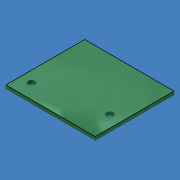
# Autodesk Inventor part: Spike PCB
Saved by Autodesk Inventor 2012 (Build 160160000, 160)
## iProperties
Shininess: 64.0
Length Units: 11269
Angle Units: 11279
Time Units: 11290
Mass Units: 11283
Length Display Precision: 3
Angle Display Precision: 2
Compacted: True
Part Number: Spike PCB
Document SubType Name: Modeling
Created: 2005-12-31
Material: Phenolic
Designer: Owner
Density: 1 g/cm^3
Density: 0.0
Volumn: 0.0
Area: 0.0
PropertySet Name: Model Information
Control State: 0
Master: False
Checked Out: False
Author: Owner
Autodesk Inventor part; units mm, degrees
ref_plane "YZ Plane" through (0, 0, 0) normal (1, 0, 0) x (0, 1, 0)
ref_plane "XZ Plane" through (0, 0, 0) normal (0, 1, 0) x (-1, 0, 0)
ref_plane "XY Plane" through (0, 0, 0) normal (0, 0, 1) x (1, 0, 0)
sketch "Sketch1" plane through (0, 0, 0) normal (0, 0, 1) x (1, 0, 0)
  line L0 (-21, 18.5) -> (21, 18.5)
  line L1 (21, 18.5) -> (21, -18.5)
  line L2 (21, -18.5) -> (-21, -18.5)
  line L3 (-21, -18.5) -> (-21, 18.5)
  line L4 (0, 0) -> (0, 18.5) construction
  line L5 (0, 0) -> (0, -18.5) construction
  line L6 (0, 0) -> (21, 0) construction
  line L7 (0, 0) -> (-21, 0) construction
  dimension "d0" = 42
  dimension "d1" = 37
  constraints: 16 end point, 4 midpoint, 3 horizontal, 2 collinear, 2 parallel, 1 perpendicular, 1 other
  measures "d0" distance of L0.start L0.end
  measures "d1" distance of L0.end L1.end
extrude "Extrusion1" add sketch "Sketch1" along normal blind 1.6
sketch "Sketch2" plane through (0, 0, 1.6) normal (0, 0, 1) x (1, 0, 0)
  line L0 (21, 18.5) -> (21, -18.5) projected
  line L1 (-21, 18.5) -> (21, 18.5) projected
  line L2 (-21, -18.5) -> (-21, 18.5) projected
  line L3 (21, -18.5) -> (-21, -18.5) projected
sketch "Sketch3" plane through (0, 0, 1.6) normal (0, 0, 1) x (1, 0, 0)
  line L0 (21, 18.5) -> (21, -18.5) projected
  line L1 (-21, -18.5) -> (-21, 18.5) projected
  line L2 (21, -18.5) -> (-21, -18.5) projected
  point P0 (-15.9, -11.65)
  point P1 (15.4, -6)
  dimension "d4" = 5.1
  dimension "d5" = 6.85
  dimension "d6" = 5.6
  dimension "d7" = 12.5
  measures "d4" distance from line of L1 point (-15.9, -11.65)
  measures "d5" distance from line of L2 point (-15.9, -11.65)
  measures "d6" distance from line of L0 point (15.4, -6)
  measures "d7" distance from line of point (15.4, -6) L2
hole "Hole1" at (-15.9, -11.65, 1.6) at (15.4, -6, 1.6) direction (0, 0, -1) diameter 3.2 end through all
body "Solid1"
